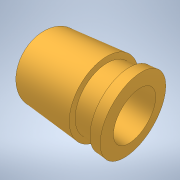
# Autodesk Inventor part: Резьбовая втулка
Saved by Autodesk Inventor 2021.1 (Build 251245010, 245A)
## iProperties
Created: 2026-05-18
Part Number: Резьбовая втулка
Material: Типовые
Document SubType Name: Modeling
Designer: Андрей Тарасов
Density: 1 g/cm^3
Appearance: По умолчанию
Author: Андрей Тарасов
Autodesk Inventor part; units mm, degrees
ref_plane "YZ Plane" through (0, 0, 0) normal (1, 0, 0) x (0, 1, 0)
ref_plane "XZ Plane" through (0, 0, 0) normal (0, 1, 0) x (-1, 0, 0)
ref_plane "XY Plane" through (0, 0, 0) normal (0, 0, 1) x (1, 0, 0)
sketch "Эскиз1" plane through (0, 0, 0) normal (0, 0, 1) x (1, 0, 0)
  line L0 (0, 1.3) -> (5, 1.3)
  line L1 (5, 1.3) -> (5, 2)
  line L2 (5, 2) -> (4.5, 2)
  line L3 (4.5, 2) -> (4.5, 1.8)
  line L4 (4.5, 1.8) -> (3.5, 1.8)
  line L5 (3.5, 1.8) -> (3.5, 2.1)
  line L6 (3.5, 2.1) -> (0, 2.1)
  line L7 (0, 2.1) -> (0, 1.3)
  line L8 (-1, 0) -> (6, 0) construction
  line L9 (0, -0.42) -> (0, 2.52) construction
  point P0 (0, 0)
  dimension "d0" = 1.3
  dimension "d1" = 2.1
  dimension "d2" = 2
  dimension "d3" = 0.5
  dimension "d4" = 5
  dimension "d5" = 0.5
  dimension "d6" = 3.5
  constraints: 16 end point, 7 perpendicular, 1 collinear, 1 horizontal
  measures "d0" distance between parallel lines of L8 L0
  measures "d1" distance between parallel lines of L8 L6
  measures "d2" distance between parallel lines of L8 L2
  measures "d3" distance between parallel lines of L0 L4
  measures "d4" distance between parallel lines of L1 L7
  measures "d5" distance between parallel lines of L1 L3
  measures "d6" distance between parallel lines of L5 L7
revolve "Вращение1" add sketch "Эскиз1" angle 360 about axis through (-10, 0, 0) along (1, 0, 0)
